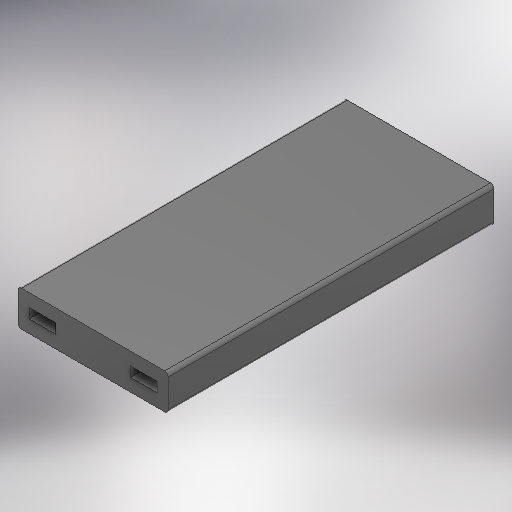
# Autodesk Inventor part: 5V_LIon_speedy
Saved by Autodesk Inventor 2026 (Build 300175050, 175E)
## iProperties
Created: 2025-06-25
Part Number: 5V_LIon_speedy
Material: Generic
Document SubType Name: Modeling
Designer: satom
Density: 1 g/cm^3
Appearance: Default
Author: satom
Autodesk Inventor part; units mm, degrees
ref_plane "YZ Plane" through (0, 0, 0) normal (1, 0, 0) x (0, 1, 0)
ref_plane "XZ Plane" through (0, 0, 0) normal (0, 1, 0) x (-1, 0, 0)
ref_plane "XY Plane" through (0, 0, 0) normal (0, 0, 1) x (1, 0, 0)
sketch "Sketch1" plane through (0, 0, 0) normal (0, 0, 1) x (1, 0, 0)
  line L0 (-32.3125, 8) -> (32.3125, 8)
  line L1 (33.9, 6.4125) -> (33.9, -6.4125)
  line L2 (32.3125, -8) -> (-32.3125, -8)
  line L3 (-33.9, -6.4125) -> (-33.9, 6.4125)
  arc A0 (-32.3125, 8) -> (-33.9, 6.4125) centre (-32.3125, 6.4125) ccw
  arc A1 (33.9, 6.4125) -> (32.3125, 8) centre (32.3125, 6.4125) ccw
  arc A2 (32.3125, -8) -> (33.9, -6.4125) centre (32.3125, -6.4125) ccw
  arc A3 (-33.9, -6.4125) -> (-32.3125, -8) centre (-32.3125, -6.4125) ccw
  dimension "d2" = 1.5875
  constraints: 8 end point, 8 point on circle, 8 tangent, 4 centre point, 3 equal radius, 2 parallel, 1 horizontal, 1 perpendicular
  measures "d2" radius of A0
extrude "Extrusion1" add sketch "Sketch1" along normal blind 147
sketch "Sketch2" plane through (0, 0, 147) normal (0, 0, 1) x (1, 0, 0)
  line L0 (-28.9, 2.25) -> (-16.9, 2.25)
  line L1 (-16.9, 2.25) -> (-16.9, -2.25)
  line L2 (-16.9, -2.25) -> (-28.9, -2.25)
  line L3 (-28.9, -2.25) -> (-28.9, 2.25)
  line L4 (-28.9, 2.25) -> (-16.9, -2.25) construction
  line L5 (-16.9, 2.25) -> (-28.9, -2.25) construction
  line L6 (16.9, 2.25) -> (28.9, 2.25)
  line L7 (28.9, 2.25) -> (28.9, -2.25)
  line L8 (28.9, -2.25) -> (16.9, -2.25)
  line L9 (16.9, -2.25) -> (16.9, 2.25)
  line L10 (16.9, 2.25) -> (28.9, -2.25) construction
  line L11 (28.9, 2.25) -> (16.9, -2.25) construction
  line L12 (-33.9, 6.4125) -> (-33.9, -6.4125) construction
  line L13 (-33.9, 0) -> (33.9, 0) construction
  line L14 (33.9, -6.4125) -> (33.9, 6.4125) construction
  point P0 (0, 0)
  point P1 (-22.9, 0)
  point P2 (22.9, 0)
  dimension "d11" = 12
  dimension "d12" = 12
  dimension "d13" = 4.5
  dimension "d14" = 4.5
  dimension "d15" = 5
  dimension "d16" = 5
  constraints: 26 end point, 6 midpoint, 4 parallel, 2 horizontal, 2 perpendicular, 2 point on line
  measures "d11" distance of L0.start L0.end
  measures "d12" distance of L6.start L6.end
  measures "d13" distance of L6.end L7.end
  measures "d14" distance of L2.end L0.start
  measures "d15" distance between parallel lines of L14 L7
  measures "d16" distance between parallel lines of L3 L12
extrude "Extrusion2" cut sketch "Sketch2" against normal blind 10
equation "\"d16\" = d15"
body "Solid1"
